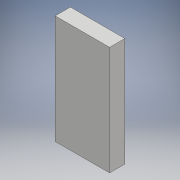
# Autodesk Inventor part: Mainboard_Placeholder
Saved by Autodesk Inventor 2017 (Build 210142000, 142)
## iProperties
Created: 2017-02-02
Part Number: Mainboard_Placeholder
Material: Generic
Document SubType Name: Modeling
Designer: Alexander Miller
Density: 1 g/cm^3
Appearance: Default
Mb_height: 50,000 mm
Mb_width: 100,000 mm
Author: Alexander Miller
Autodesk Inventor part; units mm, degrees
ref_plane "YZ Plane" through (0, 0, 0) normal (1, 0, 0) x (0, 1, 0)
ref_plane "XZ Plane" through (0, 0, 0) normal (0, 1, 0) x (-1, 0, 0)
ref_plane "XY Plane" through (0, 0, 0) normal (0, 0, 1) x (1, 0, 0)
sketch "Sketch1" plane through (0, 0, 0) normal (0, 1, 0) x (-1, 0, 0)
  line L0 (-25, 50) -> (25, 50)
  line L1 (25, 50) -> (25, -50)
  line L2 (25, -50) -> (-25, -50)
  line L3 (-25, -50) -> (-25, 50)
  point P0 (0, 0)
  point P1 (25, 0)
  point P2 (0, 50)
  dimension "d0" = 100
  dimension "d1" = 50
  constraints: 8 end point, 2 midpoint, 2 parallel, 1 horizontal, 1 horizontal alignment, 1 perpendicular, 1 vertical alignment
  measures "d0" distance of L0.end L1.end
  measures "d1" distance of L0.start L0.end
extrude "Extrusion1" add sketch "Sketch1" along normal blind 14
equation "\"d0\" = Mb_width"
equation "\"d1\" = Mb_height"
equation "\"Mb_height\" = 50"
equation "\"Mb_width\" = 100"
body "Solid1"
